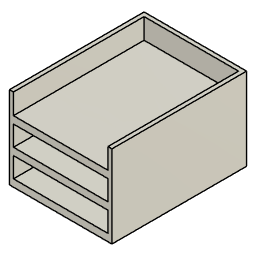
Paperstorage-V1 (Autodesk Fusion 360 design; units mm, degrees)
Autodesk Fusion 360 part; units mm, degrees
sketch "Skizze1" plane through (0, 0, 0) normal (0, 0, 1) x (1, 0, 0)
  line L0 (-15, 30) -> (240, 30)
  line L1 (240, 30) -> (240, -305)
  line L2 (240, -305) -> (-15, -305)
  line L3 (-15, -305) -> (-15, 30)
  dimension "d1" = 255
  dimension "d2" = 335
  constraint horizontal L0
  constraint vertical L1
  constraint horizontal L2
  constraint vertical L3
  measures "d1" distance of L0.start L0.end
  measures "d2" distance of L0.start L2.end
extrude "Extrusion1" add sketch "Skizze1" along normal blind 205
sketch "Skizze2" plane through (0, -305, 0) normal (0, -1, 0) x (1, 0, 0)
  line L0 (-15, 0) -> (240, 0)
  line L1 (240, 0) -> (240, 205)
  line L2 (240, 205) -> (-15, 205)
  line L3 (-15, 205) -> (-15, 0)
sketch "Skizze3" plane through (0, -305, 0) normal (0, -1, 0) x (1, 0, 0)
  line L0 (-5, 205) -> (-15, 205)
  line L1 (-15, 205) -> (-15, 0)
  line L2 (-15, 0) -> (-5, 0)
  line L3 (-5, 0) -> (-5, 205)
  line L4 (230, 0) -> (240, 0)
  line L5 (240, 0) -> (240, 205)
  line L6 (240, 205) -> (230, 205)
  line L7 (230, 205) -> (230, 0)
  line L8 (-5, 0) -> (230, 0)
  line L9 (230, 0) -> (230, 18)
  line L10 (230, 18) -> (-5, 18)
  line L11 (-5, 18) -> (-5, 0)
  line L12 (-5, 68) -> (230, 68)
  line L13 (230, 68) -> (230, 86)
  line L14 (230, 86) -> (-5, 86)
  line L15 (-5, 86) -> (-5, 68)
  line L16 (-5, 154) -> (230, 154)
  line L17 (230, 154) -> (230, 136)
  line L18 (230, 136) -> (-5, 136)
  line L19 (-5, 136) -> (-5, 154)
  line L20 (240, 205) -> (-15, 205)
  dimension "d8" = 235
  dimension "d9" = 10
  dimension "d12" = 10
  dimension "d13" = 205
  dimension "d14" = 18
  dimension "d15" = 50
  dimension "d16" = 18
  dimension "d17" = 50
  dimension "d18" = 18
  dimension "d19" = 51
  constraint horizontal L0
  constraint vertical L1
  constraint horizontal L2
  constraint vertical L3
  constraint horizontal L4
  constraint vertical L5
  constraint horizontal L6
  constraint vertical L7
  constraint horizontal L8
  constraint vertical L9
  constraint horizontal L10
  constraint vertical L11
  constraint coincident L7 L9.end
  constraint horizontal L12
  constraint vertical L13
  constraint horizontal L14
  constraint vertical L15
  constraint coincident L7 L13.end
  constraint horizontal L16
  constraint vertical L17
  constraint horizontal L18
  constraint vertical L19
  constraint coincident L7 L17.end
  constraint coincident L3 L16.start
  measures "d8" distance of L3 L7
  measures "d9" distance of L4.start L4.end
  measures "d12" distance of L1.end L2.end
  measures "d13" distance of L4.start L6.end
  measures "d14" distance of L2.end L10.end
  measures "d15" distance of L10 L12
  measures "d16" distance of L12.start L14.end
  measures "d17" distance of L14 L18
  measures "d18" distance of L16 L18
  measures "d19" distance of L16 L20
extrude "Extrusion2" cut sketch "Skizze3" against normal blind 325 contours L3 L7 L16 L20 | L3 L7 L14 L18 | L3 L7 L10 L12
